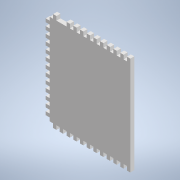
# Autodesk Inventor part: unlong2
Saved by Autodesk Inventor 2022 (Build 260153000, 153)
## iProperties
Created: 2023-05-26
Part Number: unlong2
Material: Типовые
Document SubType Name: Modeling
Designer: korsh624
Density: 1 g/cm^3
Appearance: По умолчанию
Author: korsh624
Autodesk Inventor part; units mm, degrees
ref_plane "YZ Plane" through (0, 0, 0) normal (1, 0, 0) x (0, 1, 0)
ref_plane "XZ Plane" through (0, 0, 0) normal (0, 1, 0) x (-1, 0, 0)
ref_plane "XY Plane" through (0, 0, 0) normal (0, 0, 1) x (1, 0, 0)
sketch "Эскиз1" plane through (0, 0, 0) normal (0, 0, 1) x (1, 0, 0)
  line L0 (0, 0) -> (5, 0) projected
  line L1 (5, 0) -> (5, 6) projected
  line L2 (0, 6) -> (5, 6) projected
  line L3 (0, 0) -> (0, 6) projected
  line L4 (-10, 0) -> (-5, 0) projected
  line L5 (-5, 0) -> (-5, 6) projected
  line L6 (-10, 6) -> (-5, 6) projected
  line L7 (-10, 0) -> (-10, 6) projected
  line L8 (-20, 0) -> (-15, 0) projected
  line L9 (-15, 0) -> (-15, 6) projected
  line L10 (-20, 6) -> (-15, 6) projected
  line L11 (-20, 0) -> (-20, 6) projected
  line L12 (-30, 0) -> (-25, 0) projected
  line L13 (-25, 0) -> (-25, 6) projected
  line L14 (-30, 6) -> (-25, 6) projected
  line L15 (-30, 0) -> (-30, 6) projected
  line L16 (-40, 0) -> (-35, 0) projected
  line L17 (-35, 0) -> (-35, 6) projected
  line L18 (-40, 6) -> (-35, 6) projected
  line L19 (-40, 0) -> (-40, 6) projected
  line L20 (-50, 0) -> (-45, 0) projected
  line L21 (-45, 0) -> (-45, 6) projected
  line L22 (-50, 6) -> (-45, 6) projected
  line L23 (-50, 0) -> (-50, 6) projected
  line L24 (-60, 0) -> (-55, 0) projected
  line L25 (-55, 0) -> (-55, 6) projected
  line L26 (-60, 6) -> (-55, 6) projected
  line L27 (-60, 0) -> (-60, 6) projected
  line L28 (-70, 0) -> (-65, 0) projected
  line L29 (-65, 0) -> (-65, 6) projected
  line L30 (-70, 6) -> (-65, 6) projected
  line L31 (-70, 0) -> (-70, 6) projected
  line L32 (-80, 0) -> (-75, 0) projected
  line L33 (-80, 0) -> (-75, 0) projected
  line L34 (-75, 0) -> (-75, 6) projected
  line L35 (-80, 6) -> (-75, 6) projected
  line L36 (-80, 0) -> (-80, 6) projected
  line L37 (-90, 0) -> (-85, 0) projected
  line L38 (-85, 0) -> (-85, 6) projected
  line L39 (-90, 6) -> (-85, 6) projected
  line L40 (-90, 0) -> (-90, 6) projected
  line L41 (-100, 0) -> (-100, 6) projected
  line L42 (-110, 0) -> (-105, 0) projected
  line L43 (-105, 0) -> (-105, 6) projected
  line L44 (-110, 6) -> (-105, 6) projected
  line L45 (-110, 0) -> (-110, 6) projected
  line L46 (-115, 0) -> (-110, 0) projected
  line L47 (-115, -5) -> (-115, 0) projected
  line L48 (-110, -141) -> (-105, -141) projected
  line L49 (-105, -141) -> (-105, -135) projected
  line L50 (-110, -135) -> (-105, -135) projected
  line L51 (-110, -141) -> (-110, -135) projected
  line L52 (-100, -141) -> (-95, -141) projected
  line L53 (-95, -141) -> (-95, -135) projected
  line L54 (-100, -135) -> (-95, -135) projected
  line L55 (-100, -141) -> (-100, -135) projected
  line L56 (-90, -141) -> (-85, -141) projected
  line L57 (-85, -141) -> (-85, -135) projected
  line L58 (-90, -135) -> (-85, -135) projected
  line L59 (-90, -141) -> (-90, -135) projected
  line L60 (-80, -141) -> (-75, -141) projected
  line L61 (-75, -141) -> (-75, -135) projected
  line L62 (-80, -135) -> (-75, -135) projected
  line L63 (-80, -141) -> (-80, -135) projected
  line L64 (-70, -141) -> (-65, -141) projected
  line L65 (-65, -141) -> (-65, -135) projected
  line L66 (-70, -135) -> (-65, -135) projected
  line L67 (-70, -141) -> (-70, -135) projected
  line L68 (-60, -141) -> (-55, -141) projected
  line L69 (-55, -141) -> (-55, -135) projected
  line L70 (-60, -135) -> (-55, -135) projected
  line L71 (-60, -141) -> (-60, -135) projected
  line L72 (-50, -141) -> (-45, -141) projected
  line L73 (-45, -141) -> (-45, -135) projected
  line L74 (-50, -135) -> (-45, -135) projected
  line L75 (-50, -141) -> (-50, -135) projected
  line L76 (-40, -141) -> (-35, -141) projected
  line L77 (-35, -141) -> (-35, -135) projected
  line L78 (-40, -135) -> (-35, -135) projected
  line L79 (-40, -141) -> (-40, -135) projected
  line L80 (-30, -141) -> (-25, -141) projected
  line L81 (-25, -141) -> (-25, -135) projected
  line L82 (-30, -135) -> (-25, -135) projected
  line L83 (-30, -141) -> (-30, -135) projected
  line L84 (-20, -141) -> (-15, -141) projected
  line L85 (-15, -141) -> (-15, -135) projected
  line L86 (-20, -135) -> (-15, -135) projected
  line L87 (-20, -141) -> (-20, -135) projected
  line L88 (-10, -141) -> (-5, -141) projected
  line L89 (-5, -141) -> (-5, -135) projected
  line L90 (-10, -135) -> (-5, -135) projected
  line L91 (-10, -141) -> (-10, -135) projected
  line L92 (0, -141) -> (5, -141) projected
  line L93 (5, -141) -> (5, -135) projected
  line L94 (0, -135) -> (5, -135) projected
  line L95 (0, -141) -> (0, -135) projected
  line L96 (-115, -130) -> (-115, -125) projected
  line L97 (-115, -125) -> (-121, -125) projected
  line L98 (-121, -130) -> (-121, -125) projected
  line L99 (-115, -130) -> (-121, -130) projected
  line L100 (-115, -135) -> (-115, -130) projected
  line L101 (-115, -135) -> (-110, -135) projected
  line L102 (-115, -120) -> (-115, -115) projected
  line L103 (-115, -115) -> (-121, -115) projected
  line L104 (-121, -120) -> (-121, -115) projected
  line L105 (-115, -120) -> (-121, -120) projected
  line L106 (-115, -110) -> (-115, -105) projected
  line L107 (-115, -105) -> (-121, -105) projected
  line L108 (-121, -110) -> (-121, -105) projected
  line L109 (-115, -110) -> (-121, -110) projected
  line L110 (-115, -100) -> (-115, -95) projected
  line L111 (-115, -95) -> (-121, -95) projected
  line L112 (-121, -100) -> (-121, -95) projected
  line L113 (-115, -100) -> (-121, -100) projected
  line L114 (-115, -90) -> (-115, -85) projected
  line L115 (-115, -85) -> (-121, -85) projected
  line L116 (-121, -90) -> (-121, -85) projected
  line L117 (-115, -90) -> (-121, -90) projected
  line L118 (-115, -80) -> (-115, -75) projected
  line L119 (-115, -75) -> (-121, -75) projected
  line L120 (-121, -80) -> (-121, -75) projected
  line L121 (-115, -80) -> (-121, -80) projected
  line L122 (-115, -70) -> (-115, -65) projected
  line L123 (-115, -65) -> (-121, -65) projected
  line L124 (-121, -70) -> (-121, -65) projected
  line L125 (-115, -70) -> (-121, -70) projected
  line L126 (-115, -60) -> (-115, -55) projected
  line L127 (-115, -55) -> (-121, -55) projected
  line L128 (-121, -60) -> (-121, -55) projected
  line L129 (-115, -60) -> (-121, -60) projected
  line L130 (-115, -50) -> (-115, -45) projected
  line L131 (-115, -45) -> (-121, -45) projected
  line L132 (-121, -50) -> (-121, -45) projected
  line L133 (-115, -50) -> (-121, -50) projected
  line L134 (-115, -40) -> (-115, -35) projected
  line L135 (-115, -35) -> (-121, -35) projected
  line L136 (-121, -40) -> (-121, -35) projected
  line L137 (-115, -40) -> (-121, -40) projected
  line L138 (-115, -30) -> (-115, -25) projected
  line L139 (-115, -25) -> (-121, -25) projected
  line L140 (-121, -30) -> (-121, -25) projected
  line L141 (-115, -30) -> (-121, -30) projected
  line L142 (-115, -20) -> (-115, -15) projected
  line L143 (-115, -15) -> (-121, -15) projected
  line L144 (-121, -20) -> (-121, -15) projected
  line L145 (-115, -20) -> (-121, -20) projected
  line L146 (-115, -10) -> (-115, -5) projected
  line L147 (-115, -5) -> (-121, -5) projected
  line L148 (-121, -10) -> (-121, -5) projected
  line L149 (-115, -10) -> (-121, -10) projected
  line L150 (5, 0) -> (-115, 0)
  line L151 (-115, 0) -> (-115, -135)
  line L152 (-115, -135) -> (5, -135)
  line L153 (5, -135) -> (5, 0)
  constraints: 2 end point, 1 vertical, 9 other
extrude "Выдавливание1" add sketch "Эскиз1" along normal blind 6
